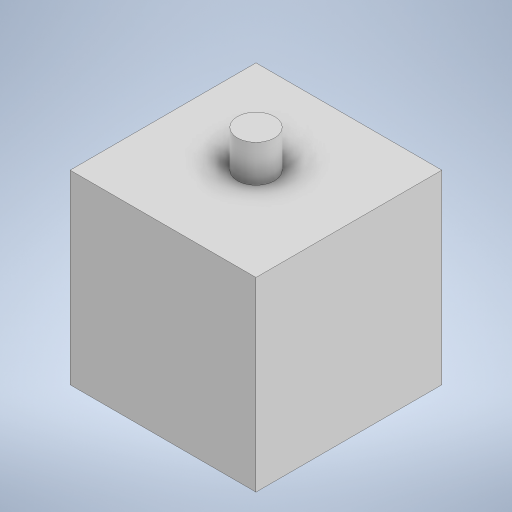
# Autodesk Inventor part: Inferior
Saved by Autodesk Inventor 2024 (Build 280153000, 153)
## iProperties
Created: 2024-10-14
Part Number: Inferior
Material: Genérico
Document SubType Name: Modeling
Designer: robof
Density: 1 g/cm^3
Appearance: Padrão
Author: robof
Autodesk Inventor part; units mm, degrees
ref_plane "YZ Plane" through (0, 0, 0) normal (1, 0, 0) x (0, 1, 0)
ref_plane "XZ Plane" through (0, 0, 0) normal (0, 1, 0) x (-1, 0, 0)
ref_plane "XY Plane" through (0, 0, 0) normal (0, 0, 1) x (1, 0, 0)
sketch "Esboço1" plane through (0, 0, 0) normal (0, 1, 0) x (-1, 0, 0)
  line L0 (0, 0) -> (50, 0)
  line L1 (50, 0) -> (50, -50)
  line L2 (50, -50) -> (0, -50)
  line L3 (0, -50) -> (0, 0)
  dimension "d0" = 50
  dimension "d1" = 50
  constraints: 8 end point, 2 parallel, 1 horizontal, 1 perpendicular
  measures "d0" distance of L1.end L2.end
  measures "d1" distance of L0.end L1.end
extrude "Extrusão1" add sketch "Esboço1" along normal blind 50
sketch "Esboço2" plane through (0, 50, 0) normal (0, 1, 0) x (1, 0, 0)
  line L0 (0, 0) -> (0, 50) projected
  line L1 (0, 25) -> (-29.0477, 25)
  line L2 (-50, 0) -> (0, 0) projected
  line L3 (-25, 0) -> (-25, 29.6188)
  circle A0 centre (-25, 25) radius 5
  dimension "d4" = 10
  constraints: 4 end point, 2 midpoint, 2 point on line, 1 centre point, 1 horizontal, 1 perpendicular
  measures "d4" diameter of A0
extrude "Extrusão2" add sketch "Esboço2" along normal blind 10 contours A0 L3 L1 | L1 L3 A0
